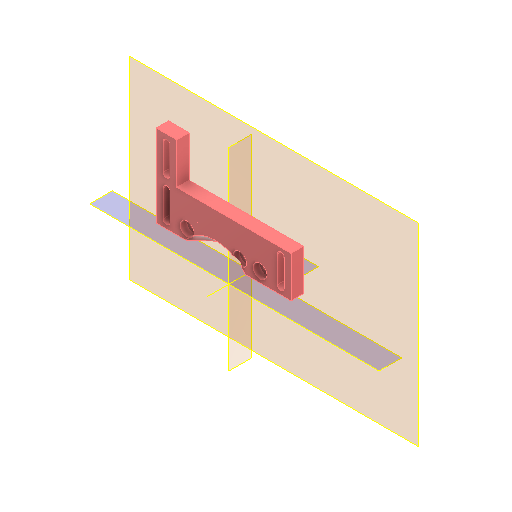
# Autodesk Inventor part: 30_Scanlens_Laseradaper_lid_v1
Saved by Autodesk Inventor 2022 (Build 260153000, 153)
## iProperties
Created: 2022-12-18
Part Number: 30_Scanlens_Laseradaper_lid_v1
Material: Generisch
Document SubType Name: Modeling
Designer: diederichbenedict
Density: 1 g/cm^3
Appearance: Glatt - Rot
Author: diederichbenedict
Autodesk Inventor part; units mm, degrees
ref_plane "YZ Plane" through (0, 0, 0) normal (1, 0, 0) x (0, 1, 0)
ref_plane "XZ Plane" through (0, 0, 0) normal (0, 1, 0) x (-1, 0, 0)
ref_plane "XY Plane" through (0, 0, 0) normal (0, 0, 1) x (1, 0, 0)
ref_plane "Arbeitsebene1" through (9.85, -10, -2.9007) normal (0, -1, 0) x (-1, 0, 0)
sketch "Skizze1" plane through (9.85, -10, -2.9007) normal (0, -1, 0) x (-1, 0, 0)
  circle A0 centre (3.75, -2.8993) radius 7 construction
  line L0 (-22.75, -4.9007) -> (-2.35, -4.9007) projected
  circle A1 centre (3.75, -2.8993) radius 6.1 construction
  line L1 (-17.6699, -15.6993) -> (-22.75, -15.6993) projected
  line L2 (22.75, -4.9007) -> (-22.75, -4.9007)
  line L3 (-22.75, -4.9007) -> (-22.75, -15.6993)
  line L4 (-22.75, -15.6993) -> (22.75, -15.6993)
  line L5 (22.75, -15.6993) -> (22.75, -4.9007)
  circle A2 centre (3.75, -2.8993) radius 5.9
  line L6 (22.75, -4.9007) -> (-22.75, -4.9007)
  line L7 (-22.75, -4.9007) -> (-22.75, -2.8993)
  line L8 (-22.75, -2.8993) -> (22.75, -2.8993)
  line L9 (22.75, -2.8993) -> (22.75, -4.9007)
  point P0 (9.85, -2.9007)
  point P1 (-22.75, -4.9007)
  point P2 (-17.6699, -15.6993)
  point P3 (-2.9578, -4.9007)
  point P4 (9.3001, -4.9007)
  point P5 (-1.8001, -4.9007)
  point P6 (-2.35, -4.9007)
  point P7 (-22.75, -4.9007)
  point P8 (-2.15, -2.8993)
  point P9 (9.65, -2.8993)
  dimension "d47" = 11.8
  constraints: 16 end point, 4 parallel, 2 horizontal, 2 perpendicular, 1 centre point, 1 coincident, 1 other
  measures "d47" diameter of A2
ref_plane "Arbeitsebene2" through (-2.9, 0, -9.8015) normal (0, 1, 0) x (0, 0, 1)
extrude "Extrusion1" add sketch "Skizze1" against normal up to surface (10 mm away) contours L7 L8 A2 L2 L0 | L0 L2 A2 L5 L4 L1 L3 | A2 L8 L2 | L2 A2 | A2 L8 L9 L2
sketch "Skizze2" plane through (-12.9, -10, 12.7985) normal (0, 0, 1) x (1, 0, 0)
  circle A0 centre (5, 5) radius 1.4 projected
  circle A1 centre (30.5801, 5) radius 1.4 projected
  circle A2 centre (40.4199, 5) radius 1.4 projected
  point P0 (12.9, 10)
hole "Bohrung1" at (-7.9, -5, 12.7985) at (17.6801, -5, 12.7985) at (27.5199, -5, 12.7985) direction (0, 0, -1) diameter 2.9 end through all counterbore diameter 6.5 counterbore depth 3
sketch "Skizze3" plane through (-12.9, -10, 12.7985) normal (0, 0, 1) x (1, 0, 0)
  circle A0 centre (30.5801, 5) radius 3.25 projected
  circle A1 centre (5, 5) radius 3.25 projected
  circle A2 centre (40.4199, 5) radius 3.25 projected
  line L0 (45.5, 10) -> (0, 10) projected
  line L1 (0, 0) -> (0, 10) projected
  line L2 (45.5, 0) -> (0, 0) projected
  line L3 (45.5, 0) -> (45.5, 10) projected
  line L4 (10, 18) -> (10, 10.0274) projected
  line L5 (3, 32.1736) -> (3, 14.9264) projected
  arc A3 (7, 32.1736) -> (3, 32.1736) centre (5, 32.1736) ccw projected
  line L6 (7, 14.9264) -> (7, 32.1736) projected
  arc A4 (3, 14.9264) -> (7, 14.9264) centre (5, 14.9264) ccw projected
  line L7 (12, 32.1736) -> (12, 20) projected
  arc A5 (12, 32.1736) -> (11.6196, 34.4497) centre (5, 32.1736) ccw projected
  arc A6 (13.5109, 37.1) -> (11.6196, 34.4497) centre (13.5109, 35.1) ccw projected
  line L8 (0.027, 37.1) -> (13.5109, 37.1) projected
  arc A7 (0.027, 37.1) -> (0, 37.0726) centre (5, 32.1736) ccw projected
  line L9 (0, 10.0274) -> (0, 37.0726) projected
  arc A8 (0, 10.0274) -> (0.027, 10) centre (5, 14.9264) ccw projected
  line L10 (9.973, 10) -> (0.027, 10) projected
  arc A9 (9.973, 10) -> (10, 10.0274) centre (5, 14.9264) ccw projected
  line L11 (10, 18) -> (10, 10.0274) projected
  arc A10 (12, 20) -> (10, 18) centre (12, 18) ccw projected
  line L12 (0, 10) -> (12.9, 10) projected
  line L13 (0, 10) -> (10, 10)
  line L14 (10, 10) -> (10, 48)
  line L15 (10, 48) -> (0, 48)
  line L16 (0, 48) -> (0, 10)
  line L17 (45.5, 0) -> (0, 0) projected
  line L18 (45.5, 0) -> (55.5, 0)
  line L19 (55.5, 0) -> (55.5, 10)
  line L20 (55.5, 10) -> (45.5, 10)
  line L21 (45.5, 10) -> (45.5, 0)
  line L22 (0, 0) -> (0, 10) projected
  line L23 (0, 0) -> (-10, 0)
  line L24 (-10, 0) -> (-10, 10)
  line L25 (-10, 10) -> (0, 10)
  line L26 (0, 10) -> (0, 0)
  line L27 (55.5, 10) -> (45.5, 10)
  line L28 (45.5, 10) -> (45.5, 20)
  line L29 (45.5, 20) -> (55.5, 20)
  line L30 (55.5, 20) -> (55.5, 10)
  line L31 (0.027, 10) -> (-9.973, 10)
  line L32 (-9.973, 10) -> (-9.973, 20)
  line L33 (-9.973, 20) -> (0.027, 20)
  line L34 (0.027, 20) -> (0.027, 10)
  line L35 (50.5, 16.5) -> (50.5, 3.5) construction
  line L36 (48.9, 16.5) -> (48.9, 3.5)
  line L37 (52.1, 3.5) -> (52.1, 16.5)
  arc A11 (52.1, 16.5) -> (48.9, 16.5) centre (50.5, 16.5) ccw
  arc A12 (48.9, 3.5) -> (52.1, 3.5) centre (50.5, 3.5) ccw
  line L38 (-4.973, 3.5) -> (-4.973, 16.5) construction
  line L39 (-3.373, 3.5) -> (-3.373, 16.5)
  line L40 (-6.573, 16.5) -> (-6.573, 3.5)
  arc A13 (-6.573, 3.5) -> (-3.373, 3.5) centre (-4.973, 3.5) ccw
  arc A14 (-3.373, 16.5) -> (-6.573, 16.5) centre (-4.973, 16.5) ccw
  line L41 (45.5, 10) -> (0, 10) projected
  line L42 (45.5, 20) -> (29.5, 20)
  line L43 (29.5, 20) -> (29.5, 10)
  line L44 (29.5, 10) -> (45.5, 10)
  line L45 (45.5, 10) -> (45.5, 20)
  line L46 (0.027, 20) -> (10, 20)
  line L47 (10, 20) -> (10, 10)
  line L48 (10, 10) -> (0.027, 10)
  line L49 (0.027, 10) -> (0.027, 20)
  line L50 (-9.973, 20) -> (0, 20)
  line L51 (0, 20) -> (0, 40)
  line L52 (0, 40) -> (-9.973, 40)
  line L53 (-9.973, 40) -> (-9.973, 20)
  line L54 (-4.9865, 23.1111) -> (-4.9865, 36.1111) construction
  line L55 (-3.3865, 23.1111) -> (-3.3865, 36.1111)
  line L56 (-6.5865, 36.1111) -> (-6.5865, 23.1111)
  arc A15 (-6.5865, 23.1111) -> (-3.3865, 23.1111) centre (-4.9865, 23.1111) ccw
  arc A16 (-3.3865, 36.1111) -> (-6.5865, 36.1111) centre (-4.9865, 36.1111) ccw
  line L57 (10, 10) -> (29.5, 10)
  line L58 (29.5, 10) -> (29.5, 20)
  line L59 (29.5, 20) -> (10, 20)
  line L60 (10, 20) -> (10, 10)
  point P0 (0, 10)
  point P1 (45.5, 10)
  point P2 (0, 37.0726)
  point P3 (0, 20)
  point P4 (-9.973, 10)
  point P5 (0, 10)
  point P6 (45.5, 10)
  point P7 (50.5, 10)
  point P8 (-4.973, 10)
  point P9 (45.5, 10)
  point P10 (10, 20)
  point P11 (29.5, 10)
  point P12 (45.5, 10)
  point P13 (-4.9865, 29.6111)
  point P14 (12, 20)
  point P15 (10, 10.0274)
  point P16 (10, 10)
  point P17 (10, 20)
  dimension "d9" = 38
  dimension "d10" = 10
  dimension "d11" = 10
  dimension "d12" = 10
  dimension "d13" = 10
  dimension "d30" = 10
  dimension "d31" = 10
  dimension "d32" = 10
  dimension "d33" = 10
  dimension "d34" = 6.5
  dimension "d35" = 3.2
  dimension "d36" = 6.5
  dimension "d37" = 3.2
  dimension "d49" = 20
  dimension "d50" = 6.5
  dimension "d51" = 3.2
  constraints: 96 end point, 22 parallel, 12 point on circle, 12 tangent, 10 perpendicular, 9 horizontal, 6 centre point, 5 midpoint, 1 point on line, 2 other
  measures "d9" distance of L14.end L13.end
  measures "d10" distance of L20.end L19.end
  measures "d11" distance of L19.end L18.end
  measures "d12" distance of L24.end L25.end
  measures "d13" distance of L23.end L24.end
  measures "d30" distance of L28.end L29.end
  measures "d31" distance of L27.end L28.end
  measures "d32" distance of L32.end L33.end
  measures "d33" distance of L31.end L32.end
  measures "d34" distance of point (50.5, 10) L35.end
  measures "d35" diameter of A12
  measures "d36" distance of point (-4.973, 10) L38.end
  measures "d37" diameter of A14
  measures "d49" distance of L51.end L50.end
  measures "d50" distance of point (-4.986, 29.611) L54.end
  measures "d51" diameter of A16
ref_plane "Arbeitsebene4" through (-15.175, -1.3586, -0.0015) normal (0, 0, -1) x (0, 1, 0)
ref_plane "Arbeitsebene5" through (-39.4, -44, 2.8735) normal (0, 0, 1) x (1, 0, 0)
extrude "Extrusion2" add sketch "Skizze3" against normal blind 6 contours L20 L36 A12 L37 L19 L18 L3 | L28 L29 L30 L20 L37 A11 L36 | L0 L43 L42 L28 | L0 L14 L4 A10 L59 L43 | L23 L24 L25 L40 A13 L39 L1 | A10 L14 L59 | L16 A8 L0 | L25 L39 A14 L40 L32 L33 L9 L16 | L0 L34 L46 L5 A4 L6 L14 L4 A9 | A8 L9 L33 L34 | L6 A4 L5 L46 | L33 L53 L52 L16 L9
ref_plane "Arbeitsebene3" through (24.5, -13.25, 2.8735) normal (0, 0, 1) x (-1, 0, 0)
ref_plane "Arbeitsebene6" through (5.9204, -16.8251, 5.7985) normal (1, 0, 0) x (0, 0, 1)
ref_plane "Arbeitsebene7" through (15.7, -24.5751, 5.7985) normal (0, -1, 0) x (-1, 0, 0)
sketch "Skizze7" plane through (5.9204, -16.8251, 5.7985) normal (1, 0, 0) x (0, 0, 1)
  line L0 (-16.7435, 4.5) -> (15.5561, 4.5)
  line L1 (15.5561, 4.5) -> (15.5561, -20.5)
  line L2 (15.5561, -20.5) -> (-16.7435, 4.5)
  circle A0 centre (-4.875, 4.5) radius 4.0105 projected
  point P0 (-5.7985, -16.8251)
  point P1 (-2.875, 4.5)
  dimension "d52" = 25
  constraints: 6 end point, 1 horizontal, 1 perpendicular, 1 point on line
  measures "d52" distance of L0.end L1.end
revolve "Umdrehung1" cut sketch "Skizze7" angle 360 about axis through (5.9204, -21.3251, -10.945) along (0, 0, 1) picked at (-5.6344, 3.3998) contours A0 L0 | L0 L1 L2 A0
ref_plane "Arbeitsebene8" through (5.9204, -8.9, -5.8803) normal (1, 0, 0) x (0, 1, 0)
sketch "Skizze8" plane through (5.9204, -8.9, -5.8803) normal (1, 0, 0) x (0, 1, 0)
  line L0 (1.9, 0.8788) -> (-0.1, 0.8788) projected
  arc A0 (1.9, 0.8788) -> (1.9, 10.8788) centre (0.4717, 5.8788) ccw projected
  line L1 (-0.1, 10.8788) -> (1.9, 10.8788) projected
  line L2 (-0.1, 0.8788) -> (-0.1, 10.8788) projected
  arc A1 (1.9139, 0.7788) -> (1.9139, 10.9788) centre (0.4717, 5.8788) ccw
  line L3 (1.9139, 0.7788) -> (-0.2, 0.7788)
  line L4 (-0.2, 0.7788) -> (-0.2, 10.9788)
  line L5 (-0.2, 10.9788) -> (1.9139, 10.9788)
  point P0 (8.9, 5.8803)
  dimension "d54" = 0.1
  constraints: 6 end point, 2 point on circle, 1 centre point, 3 other
  measures "d54" radial gap between concentric circles of A0 A1
extrude "Extrusion5" cut sketch "Skizze8" along normal mid plane 12.5 contours L0 L2 L1 A0 | L3 L4 L5 A1
sketch "Skizze9" plane through (-12.9, 0, -0.0015) normal (0, 1, 0) x (1, 0, 0)
  line L0 (10, -6.8) -> (45.5, -6.8) projected
  line L1 (45.5, 0) -> (45.5, -6.8) projected
  line L2 (0, 0) -> (45.5, 0) projected
  line L3 (0, -6.8) -> (0, 0) projected
  line L4 (0, -6.8) -> (9.973, -6.8) projected
  line L5 (9.973, -6.8) -> (9.973, -12.8) projected
  line L6 (10, -12.8) -> (9.973, -12.8) projected
  line L7 (18.8204, 5.56) -> (18.8204, -15.86) projected
  circle A0 centre (18.8204, 0) radius 2.5
  line L8 (10, -12.8) -> (10, -6.8) projected
  point P0 (12.9, -0.0015)
  dimension "d57" = 5
  constraints: 2 point on line, 1 centre point
  measures "d57" diameter of A0
extrude "Extrusion6" cut sketch "Skizze9" against normal through all contours A0 L2 L7 | L7 L2 A0 | L7 A0 L2 | L2 A0 L7
